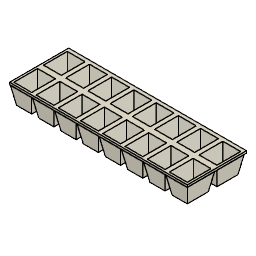
ice cube tray (Autodesk Fusion 360 design; units mm, degrees)
part number: 2025-11-21-18-31-51-986
Autodesk Fusion 360 part; units mm, degrees
sketch "Sketch1" plane through (0, 0, 0) normal (0, 1, 0) x (1, 0, 0)
  line L0 (60, -20) -> (-60, -20)
  line L1 (-60, -20) -> (-60, 20)
  line L2 (-60, 20) -> (60, 20)
  line L3 (60, 20) -> (60, -20)
  line L4 (60, -20) -> (-60, 20) construction
  line L5 (-60, -20) -> (60, 20) construction
  dimension "d1" = 120
  dimension "d2" = 40
  constraint horizontal L0
  constraint perpendicular L0 L1
  constraint parallel L0 L2
  constraint parallel L1 L3
  constraint coincident L4 origin
  constraint coincident L5 origin
  measures "d1" distance of L1.end L2.end
  measures "d2" distance of L0.end L1.end
extrude "Extrude1" add sketch "Sketch1" along normal blind 15
sketch "Sketch2" plane through (0, 15, 0) normal (0, 1, 0) x (-1, 0, 0)
  line L0 (-60, -20) -> (60, -20)
  line L1 (60, -20) -> (60, 20)
  line L2 (60, 20) -> (-60, 20)
  line L3 (-60, 20) -> (-60, -20)
  line L4 (58.5, 18.5) -> (46.5, 18.5)
  line L5 (46.5, 18.5) -> (46.5, 2.5)
  line L6 (46.5, 2.5) -> (58.5, 2.5)
  line L7 (58.5, 2.5) -> (58.5, 18.5)
  dimension "d5" = 12
  dimension "d6" = 16
  dimension "d7" = 1.5
  dimension "d8" = 1.5
  constraint horizontal L4
  constraint vertical L5
  constraint horizontal L6
  constraint vertical L7
  measures "d5" distance of L4.start L4.end
  measures "d6" distance of L4.start L6.end
  measures "d7" distance of L1 L7
  measures "d8" distance of L2 L4
extrude "1st ice cube" cut sketch "Sketch2" against normal blind 12 draft -10 contours L4 L5 L6 L7
pattern_linear "R-Pattern1" count 8 spacing 15 along (1, 0, 0) count 2 spacing 20 along (0, 0, -1) of "1st ice cube"
shell "Shell2" thickness 1.5 removed faces 5 at (-60, 10, 6.6667) at (-20, 5, -20) at (20, 0, 6.6667) at (60, 10, -6.6667) at (20, 5, 20)
